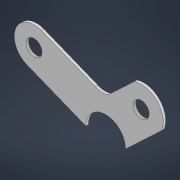
# Autodesk Inventor part: FixaçãoTanque_2
Saved by Autodesk Inventor 2022 (Build 260153000, 153)
## iProperties
Created: 2022-05-19
Part Number: FixaçãoTanque_2
Material: Genérico
Document SubType Name: Modeling
Designer: Gugarauj07
Density: 1 g/cm^3
Appearance: Padrão
Author: Gugarauj07
Autodesk Inventor part; units mm, degrees
ref_plane "YZ Plane" through (0, 0, 0) normal (1, 0, 0) x (0, 1, 0)
ref_plane "XZ Plane" through (0, 0, 0) normal (0, 1, 0) x (-1, 0, 0)
ref_plane "XY Plane" through (0, 0, 0) normal (0, 0, 1) x (1, 0, 0)
sketch "Esboço1" plane through (0, 0, 0) normal (0, 0, 1) x (1, 0, 0)
  arc A0 (0, 12.7) -> (-12.7, 0) centre (0, 0) ccw
  line L0 (-12.7, 0) -> (-50.5327, 15.1125)
  arc A1 (-41.1105, 38.7003) -> (-50.5327, 15.1125) centre (-45.8216, 26.9064) ccw
  line L1 (-41.1105, 38.7003) -> (-6.6683, 24.9421)
  circle A2 centre (-45.8216, 26.9064) radius 5.08
  arc A3 (12.7, 0) -> (0, 12.7) centre (0, 0) ccw
  line L2 (12.7, 0) -> (35.7944, 21.7352)
  arc A4 (35.7944, 21.7352) -> (18.3865, 40.2318) centre (22.7584, 26.9064) ccw
  line L3 (18.3865, 40.2318) -> (1.7519, 24.5762)
  circle A5 centre (22.7584, 26.9064) radius 5.08
  line L4 (0, 0) -> (0, 57.6178)
  arc A6 (-6.6683, 24.9421) -> (1.7519, 24.5762) centre (-2.0506, 34.1381) ccw
  dimension "d2" = 12.7
  dimension "d3" = 10.16
  dimension "d5" = 26.9064
  dimension "d6" = 12.7
  dimension "d10" = 25.4
  dimension "d11" = 114.962
  dimension "d15" = 26.9064
  dimension "d16" = 25.4
  dimension "d17" = 25.4
  dimension "d18" = 45.8216
  dimension "d19" = 40.7395
  dimension "d20" = 22.7584
  dimension "d21" = 7.62
  dimension "d22" = 12.7
  dimension "d23" = 7.62
  constraints: 10 end point, 10 point on circle, 7 centre point, 3 coincident, 2 parallel, 1 tangent, 1 vertical, 5 other
  measures "d2" radius of A1
  measures "d3" diameter of A2
  measures "d5" vertical distance of L0.start A1.centre
  measures "d6" radius of A0
  measures "d10" distance of L2.start L0.start
  measures "d11" angle of L3 L1
  measures "d15" vertical distance of L2.start A4.centre
  measures "d16" distance between parallel lines of L2 L3
  measures "d17" distance between parallel lines of L0 L1
  measures "d18" distance from line of L4 A1.centre
  measures "d19" distance of L0.start L0.end
  measures "d20" distance from line of L4 A4.centre
  measures "d21" radial gap between concentric circles of A1 A2
  measures "d22" distance from line of L2 A5.centre
  measures "d23" distance edge to line of A5 L3
extrude "Extrusão1" add sketch "Esboço1" along normal blind 1.6
